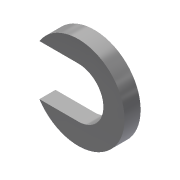
# Autodesk Inventor part: Special_Key
Saved by Autodesk Inventor 2022 Beta2 (Build 260130000, 130) ContinuousBuild 0
## iProperties
Created: 2006-01-18
Part Number: Special_Key
Document SubType Name: Modeling
Designer: PMiller
Material: Steel, Mild
Density: 7.86 g/cm^3
Appearance: Steel
Author: PMiller
Autodesk Inventor part; units mm, degrees
ref_plane "YZ Plane" through (0, 0, 0) normal (1, 0, 0) x (0, 1, 0)
ref_plane "XZ Plane" through (0, 0, 0) normal (0, 1, 0) x (-1, 0, 0)
ref_plane "XY Plane" through (0, 0, 0) normal (0, 0, 1) x (1, 0, 0)
sketch "Sketch1" plane through (0, 0, 0) normal (0, 0, 1) x (1, 0, 0)
  circle A0 centre (0, 0) radius 9.1281
  dimension "d0" = 18.2563
  constraints: 1 centre point, 1 coincident
  measures "d0" diameter of A0
extrude "Extrusion1" add sketch "Sketch1" along normal mid plane 3.175
sketch "Sketch2" plane through (0, 0, 1.5875) normal (0, 0, 1) x (1, 0, 0)
  circle A0 centre (0, 0) radius 9.1281 projected
  line L0 (-7.6624, 4.9609) -> (0, 4.9609)
  arc A1 (0, -4.9609) -> (0, 4.9609) centre (0, 0) ccw
  line L1 (0, -4.9609) -> (-7.6624, -4.9609)
  dimension "d4" = 9.9219
  constraints: 4 end point, 4 point on circle, 2 tangent, 1 centre point, 1 coincident, 1 horizontal, 1 parallel
  measures "d4" distance between parallel lines of L1 L0
extrude "Extrusion2" cut sketch "Sketch2" against normal through all contours L0 A1 L1 A0 picked at (-3.0226, 0.3489)
body "Solid1"
